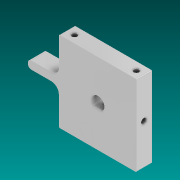
# Autodesk Inventor part: bevestegingsKoppeling axis4_5 10mm
Saved by Autodesk Inventor 2020 (Build 240168000, 168)
## iProperties
Created: 2020-05-27
Part Number: bevestegingsKoppeling axis4_5 10mm
Material: Aluminum 6061
Document SubType Name: Modeling
Designer: stefa
Density: 2.7 g/cm^3
Appearance: Aluminum - Polished
Author: stefa
Autodesk Inventor part; units mm, degrees
note: some values were not read from the file. Chosen so that the rebuilt part matches the saved one: direction of "Hole2"; direction of "Hole3".
ref_plane "YZ Plane" through (0, 0, 0) normal (1, 0, 0) x (0, 1, 0)
ref_plane "XZ Plane" through (0, 0, 0) normal (0, 1, 0) x (-1, 0, 0)
ref_plane "XY Plane" through (0, 0, 0) normal (0, 0, 1) x (1, 0, 0)
sketch "Sketch1" plane through (0, 0, 0) normal (0, 0, 1) x (1, 0, 0)
  line L0 (-25, -26) -> (25, -26)
  line L1 (25, -26) -> (25, 26)
  line L2 (25, 26) -> (-25, 26)
  line L3 (-25, 26) -> (-25, -26)
  line L4 (-25, -26) -> (25, 26) construction
  line L5 (25, -26) -> (-25, 26) construction
  circle A0 centre (0, 0) radius 4
  line L6 (-2.6458, -3) -> (2.6458, -3)
  line L7 (-45, 2.5) -> (-5, 2.5)
  line L8 (-5, 2.5) -> (-5, -2.5)
  line L9 (-5, -2.5) -> (-45, -2.5)
  line L10 (-45, -2.5) -> (-45, 2.5)
  line L11 (-45, 2.5) -> (-5, -2.5) construction
  line L12 (-5, 2.5) -> (-45, -2.5) construction
  point P0 (-25, 0)
  point P1 (-25, -2.5)
  point P2 (-25, 2.5)
  dimension "d0" = 50
  dimension "d1" = 52
  dimension "d2" = 8
  dimension "d39" = 3
  dimension "d40" = 20
  dimension "d41" = 5
  constraints: 26 end point, 5 midpoint, 5 parallel, 3 horizontal, 2 perpendicular, 2 point on circle, 1 centre point, 1 coincident
  measures "d0" distance of L2.end L1.end
  measures "d1" distance of L1.end L0.end
  measures "d2" diameter of A0
  measures "d39" distance from line of L6 point (0, 0)
  measures "d40" distance between parallel lines of L10 L3
  measures "d41" distance between parallel lines of L9 L7
extrude "Extrusion1" add sketch "Sketch1" along normal blind 10 contours L3 L9 L8 L7 L2 L1 L0 | L9 L10 L7 L3 | L3 L7 L8 L9 | L6 A0 picked at (-0.6179, -3.1815)
sketch "Sketch2" plane through (-25, -26, 0) normal (0, -1, 0) x (1, 0, 0)
  line L0 (0, 0) -> (0, 10) projected
  line L1 (50, 0) -> (50, 10) projected
  line L2 (0, 0) -> (50, 0) projected
  point P0 (25, 0)
  point P1 (0, 5)
  point P2 (45, 5)
  point P3 (25, 5)
  point P4 (5, 5)
  point P5 (0, 5)
  point P6 (50, 5)
  point P7 (25, 0)
  dimension "d19" = 5
  dimension "d20" = 5
  constraints: 4 horizontal alignment, 4 midpoint, 1 vertical alignment
  measures "d19" distance from line of L1 point (45, 5)
  measures "d20" distance from line of point (5, 5) L0
hole "Hole1" at (20, -26, 5) at (-20, -26, 5) direction (0, 1, 0) diameter 3.242 depth 15 tip angle 118 countersink diameter 4 countersink angle 90 thread size "M4x0.7" class "6H" standard "ANSI Metric M Profile"
fillet "Fillet2" radius 0.5 8 edges at (0, 4, 10) (-25, -26, 5) (25, -26, 5) (25, 26, 5) (-25, 26, 5) (0, 4, 0) (0, -3, 10) (0, -3, 0)
hole "Hole2" at (0, -26, 5) direction (0, 1, 0) diameter 3.242 end up to surface countersink diameter 4 countersink angle 90 thread size "M4x0.7" class "6H" standard "ANSI Metric M Profile"
mirror "Mirror1" about plane through (0, 0, 0) normal (0, 1, 0) of "Hole1"
sketch "Sketch3" plane through (25, -25.5, 0.5) normal (1, 0, 0) x (0, 0, -1)
  line L0 (-9.5, 51) -> (0.5, 51) projected
  point P0 (0.5, 25.5)
  point P1 (-4.5, 25.5)
  point P2 (-4.5, 51)
  point P3 (-9, 51)
  point P4 (0, 51)
  constraints: 1 horizontal alignment, 1 midpoint, 1 vertical alignment
hole "Hole3" at (25, 0, 5) direction (-1, 0, 0) diameter 3.242 end up to surface countersink diameter 4 countersink angle 90 thread size "M4x0.7" class "6H" standard "ANSI Metric M Profile"
fillet "Fillet3" radius 2 2 edges at (-45, 2.5, 5) (-45, -2.5, 5)
fillet "Fillet4" radius 5 2 edges at (-25, -2.5, 5) (-25, 2.5, 5)
body "Solid1"
